Autodesk Fusion 360 part; units mm, degrees
(part 3 of 4)
  spline S773 degree 3 poles (-4.0952, -2.1163) (-4.5357, -1.9459) (-4.7047, -1.6279) (-4.6025, -1.1626) knots 0 0 0 0 1 1 1 1
  spline S774 degree 3 poles (-4.6025, -1.1626) (-4.3484, -0.6512) (-3.9899, -0.225) (-3.527, 0.1159) knots 0 0 0 0 1 1 1 1
  spline S775 degree 3 poles (-3.527, 0.1159) (-2.8898, 0.6509) (-2.1728, 1.0365) (-1.376, 1.2726) knots 0 0 0 0 1 1 1 1
  spline S776 degree 3 poles (-1.1325, 0.6232) (-2.2555, 0.3285) (-3.2092, -0.2533) (-3.9938, -1.122) knots 0 0 0 0 1 1 1 1
  spline S777 degree 3 poles (-3.9938, -1.122) (-4.1157, -1.269) (-4.1969, -1.4313) (-4.2373, -1.609) knots 0 0 0 0 1 1 1 1
  spline S778 degree 3 poles (-4.2373, -1.609) (-4.1708, -1.7027) (-4.0829, -1.7636) (-3.9735, -1.7916) knots 0 0 0 0 1 1 1 1
  spline S779 degree 3 poles (-3.9735, -1.7916) (-3.69, -1.836) (-3.4194, -1.7954) (-3.1617, -1.6699) knots 0 0 0 0 1 1 1 1
  spline S780 degree 3 poles (-3.1617, -1.6699) (-2.1944, -1.1222) (-1.3624, -0.4119) (-0.6657, 0.4609) knots 0 0 0 0 1 1 1 1
  spline S781 degree 3 poles (-0.6657, 0.4609) (-0.6205, 0.512) (-0.6138, 0.5594) (-0.6454, 0.6029) knots 0 0 0 0 1 1 1 1
  spline S782 degree 3 poles (-0.6454, 0.6029) (-0.8072, 0.6232) (-0.9695, 0.63) (-1.1325, 0.6232) knots 0 0 0 0 1 1 1 1
  spline S783 degree 3 poles (-14.7693, 1.2726) (-14.412, 1.3072) (-14.0737, 1.2463) (-13.7546, 1.09) knots 0 0 0 0 1 1 1 1
  spline S784 degree 3 poles (-13.7546, 1.09) (-13.6135, 0.9404) (-13.5932, 0.7713) (-13.6938, 0.5826) knots 0 0 0 0 1 1 1 1
  spline S785 degree 3 poles (-13.6938, 0.5826) (-13.9508, 0.1629) (-14.2688, -0.2092) (-14.6475, -0.5335) knots 0 0 0 0 1 1 1 1
  spline S786 degree 3 poles (-14.6475, -0.5335) (-15.0534, -0.8582) (-15.4592, -1.1828) (-15.8651, -1.5075) knots 0 0 0 0 1 1 1 1
  spline S787 degree 3 poles (-15.8651, -1.5075) (-16.2645, -1.7884) (-16.6974, -2.0049) (-17.1638, -2.1569) knots 0 0 0 0 1 1 1 1
  spline S788 degree 3 poles (-17.1638, -2.1569) (-17.7724, -2.2659) (-18.1377, -2.0224) (-18.2597, -1.4264) knots 0 0 0 0 1 1 1 1
  spline S789 degree 3 poles (-18.2597, -1.4264) (-18.1127, -0.9302) (-17.8422, -0.5108) (-17.4479, -0.1682) knots 0 0 0 0 1 1 1 1
  spline S790 degree 3 poles (-17.4479, -0.1682) (-16.6732, 0.537) (-15.7804, 1.0173) (-14.7693, 1.2726) knots 0 0 0 0 1 1 1 1
  spline S791 degree 3 poles (-14.8099, 0.5826) (-16.001, 0.2541) (-16.9818, -0.3953) (-17.7523, -1.3655) knots 0 0 0 0 1 1 1 1
  spline S792 degree 3 poles (-17.7523, -1.3655) (-17.916, -1.5781) (-17.8686, -1.7202) (-17.6103, -1.7916) knots 0 0 0 0 1 1 1 1
  spline S793 degree 3 poles (-17.6103, -1.7916) (-17.4615, -1.8187) (-17.3127, -1.8187) (-17.1638, -1.7916) knots 0 0 0 0 1 1 1 1
  spline S794 degree 3 poles (-17.1638, -1.7916) (-16.7697, -1.6554) (-16.4044, -1.4661) (-16.068, -1.2234) knots 0 0 0 0 1 1 1 1
  spline S795 degree 3 poles (-16.068, -1.2234) (-15.3561, -0.7146) (-14.7067, -0.1328) (-14.1199, 0.5218) knots 0 0 0 0 1 1 1 1
  spline S796 degree 3 poles (-14.1199, 0.5218) (-14.3424, 0.5806) (-14.5724, 0.6009) (-14.8099, 0.5826) knots 0 0 0 0 1 1 1 1
  spline S797 degree 3 poles (16.9284, 1.2726) (17.2847, 1.3072) (17.6232, 1.2463) (17.943, 1.09) knots 0 0 0 0 1 1 1 1
  spline S798 degree 3 poles (17.943, 1.09) (18.0185, 1.042) (18.0591, 0.9743) (18.0648, 0.887) knots 0 0 0 0 1 1 1 1
  spline S799 degree 3 poles (18.0648, 0.887) (18.0441, 0.7035) (17.9832, 0.5344) (17.8821, 0.3797) knots 0 0 0 0 1 1 1 1
  spline S800 degree 3 poles (17.8821, 0.3797) (17.6484, 0.0646) (17.3846, -0.2263) (17.0907, -0.4929) knots 0 0 0 0 1 1 1 1
  spline S801 degree 3 poles (17.0907, -0.4929) (16.6849, -0.8176) (16.279, -1.1423) (15.8731, -1.4669) knots 0 0 0 0 1 1 1 1
  spline S802 degree 3 poles (15.8731, -1.4669) (15.4003, -1.8421) (14.8658, -2.0788) (14.27, -2.1772) knots 0 0 0 0 1 1 1 1
  spline S803 degree 3 poles (14.27, -2.1772) (13.5646, -2.0944) (13.3211, -1.7156) (13.5395, -1.0408) knots 0 0 0 0 1 1 1 1
  spline S804 degree 3 poles (13.5395, -1.0408) (14.2059, -0.0906) (15.0785, 0.6061) (16.1572, 1.0494) knots 0 0 0 0 1 1 1 1
  spline S805 degree 3 poles (16.1572, 1.0494) (16.4142, 1.1438) (16.6711, 1.2182) (16.9284, 1.2726) knots 0 0 0 0 1 1 1 1
  spline S806 degree 3 poles (16.8878, 0.5826) (16.6881, 0.5291) (16.4852, 0.4682) (16.279, 0.4) knots 0 0 0 0 1 1 1 1
  spline S807 degree 3 poles (16.279, 0.4) (15.2944, -0.0031) (14.4896, -0.6321) (13.8642, -1.4872) knots 0 0 0 0 1 1 1 1
  spline S808 degree 3 poles (13.8642, -1.4872) (13.8341, -1.566) (13.8406, -1.6404) (13.8844, -1.7105) knots 0 0 0 0 1 1 1 1
  spline S809 degree 3 poles (13.8844, -1.7105) (14.1799, -1.8416) (14.4774, -1.8416) (14.7773, -1.7105) knots 0 0 0 0 1 1 1 1
  spline S810 degree 3 poles (14.7773, -1.7105) (15.1357, -1.5382) (15.4738, -1.3352) (15.792, -1.1017) knots 0 0 0 0 1 1 1 1
  spline S811 degree 3 poles (15.792, -1.1017) (16.4174, -0.6385) (16.9925, -0.1177) (17.5169, 0.4609) knots 0 0 0 0 1 1 1 1
  spline S812 degree 3 poles (17.5169, 0.4609) (17.5364, 0.4994) (17.5433, 0.5399) (17.5372, 0.5826) knots 0 0 0 0 1 1 1 1
  spline S813 degree 3 poles (17.5372, 0.5826) (17.3208, 0.5826) (17.1041, 0.5826) (16.8878, 0.5826) knots 0 0 0 0 1 1 1 1
  spline S814 degree 3 poles (25.6543, 1.1914) (25.6815, 1.0697) (25.7083, 0.9479) (25.7355, 0.8262) knots 0 0 0 0 1 1 1 1
  spline S815 degree 3 poles (25.7355, 0.8262) (25.7331, 0.8041) (25.7197, 0.7906) (25.6949, 0.7856) knots 0 0 0 0 1 1 1 1
  spline S816 degree 3 poles (25.6949, 0.7856) (25.6547, 0.9182) (25.6413, 1.0535) (25.6543, 1.1914) knots 0 0 0 0 1 1 1 1
  spline S817 degree 3 poles (10.8405, 1.0697) (10.9899, 1.0764) (11.1388, 1.0696) (11.287, 1.0494) knots 0 0 0 0 1 1 1 1
  spline S818 degree 3 poles (11.287, 1.0494) (11.4051, 1.044) (11.5, 0.9966) (11.5711, 0.9073) knots 0 0 0 0 1 1 1 1
  spline S819 degree 3 poles (11.5711, 0.9073) (11.4379, 0.7542) (11.2756, 0.6393) (11.084, 0.5623) knots 0 0 0 0 1 1 1 1
  spline S820 degree 3 poles (11.084, 0.5623) (10.6031, 0.3564) (10.1161, 0.3293) (9.6229, 0.4812) knots 0 0 0 0 1 1 1 1
  spline S821 degree 3 poles (9.6229, 0.4812) (9.9951, 0.7552) (10.401, 0.9514) (10.8405, 1.0697) knots 0 0 0 0 1 1 1 1
  spline S822 degree 3 poles (10.7999, 0.8667) (10.5828, 0.7924) (10.3665, 0.7045) (10.1506, 0.6029) knots 0 0 0 0 1 1 1 1
  spline S823 degree 3 poles (10.1506, 0.6029) (10.5418, 0.5621) (10.9071, 0.6432) (11.2464, 0.8464) knots 0 0 0 0 1 1 1 1
  spline S824 degree 3 poles (11.2464, 0.8464) (11.0982, 0.8667) (10.9493, 0.8734) (10.7999, 0.8667) knots 0 0 0 0 1 1 1 1
  spline S825 degree 3 poles (-1.3354, 0.7856) (-1.0645, 0.7923) (-0.7939, 0.7856) (-0.5237, 0.7653) knots 0 0 0 0 1 1 1 1
  spline S826 degree 3 poles (-0.5237, 0.7653) (-0.4472, 0.7565) (-0.3795, 0.7294) (-0.3207, 0.6841) knots 0 0 0 0 1 1 1 1
  spline S827 degree 3 poles (-0.3207, 0.6841) (-0.5262, 0.3433) (-0.763, 0.0254) (-1.031, -0.2697) knots 0 0 0 0 1 1 1 1
  spline S828 degree 3 poles (-1.031, -0.2697) (-1.5589, -0.7979) (-2.1339, -1.2646) (-2.7559, -1.6699) knots 0 0 0 0 1 1 1 1
  spline S829 degree 3 poles (-2.7559, -1.6699) (-3.1548, -1.9247) (-3.5877, -2.0194) (-4.0546, -1.954) knots 0 0 0 0 1 1 1 1
  spline S830 degree 3 poles (-4.0546, -1.954) (-4.485, -1.8081) (-4.5594, -1.5579) (-4.2779, -1.2031) knots 0 0 0 0 1 1 1 1
  spline S831 degree 3 poles (-4.2779, -1.2031) (-3.6287, -0.4193) (-2.8373, 0.1827) (-1.9036, 0.6029) knots 0 0 0 0 1 1 1 1
  spline S832 degree 3 poles (-1.9036, 0.6029) (-1.7093, 0.6647) (-1.52, 0.7256) (-1.3354, 0.7856) knots 0 0 0 0 1 1 1 1
  spline S833 degree 3 poles (-1.1325, 0.6232) (-2.2555, 0.3285) (-3.2092, -0.2533) (-3.9938, -1.122) knots 0 0 0 0 1 1 1 1
  spline S834 degree 3 poles (-3.9938, -1.122) (-4.1157, -1.269) (-4.1969, -1.4313) (-4.2373, -1.609) knots 0 0 0 0 1 1 1 1
  spline S835 degree 3 poles (-4.2373, -1.609) (-4.1708, -1.7027) (-4.0829, -1.7636) (-3.9735, -1.7916) knots 0 0 0 0 1 1 1 1
  spline S836 degree 3 poles (-3.9735, -1.7916) (-3.69, -1.836) (-3.4194, -1.7954) (-3.1617, -1.6699) knots 0 0 0 0 1 1 1 1
  spline S837 degree 3 poles (-3.1617, -1.6699) (-2.1944, -1.1222) (-1.3624, -0.4119) (-0.6657, 0.4609) knots 0 0 0 0 1 1 1 1
  spline S838 degree 3 poles (-0.6657, 0.4609) (-0.6205, 0.512) (-0.6138, 0.5594) (-0.6454, 0.6029) knots 0 0 0 0 1 1 1 1
  spline S839 degree 3 poles (-0.6454, 0.6029) (-0.8072, 0.6232) (-0.9695, 0.63) (-1.1325, 0.6232) knots 0 0 0 0 1 1 1 1
  spline S840 degree 3 poles (-14.7693, 0.7856) (-14.4789, 0.8022) (-14.1948, 0.7684) (-13.917, 0.6841) knots 0 0 0 0 1 1 1 1
  spline S841 degree 3 poles (-13.917, 0.6841) (-13.8984, 0.6673) (-13.8849, 0.647) (-13.8764, 0.6232) knots 0 0 0 0 1 1 1 1
  spline S842 degree 3 poles (-13.8764, 0.6232) (-13.9748, 0.4127) (-14.1033, 0.2233) (-14.262, 0.055) knots 0 0 0 0 1 1 1 1
  spline S843 degree 3 poles (-14.262, 0.055) (-14.9117, -0.568) (-15.6084, -1.1294) (-16.3521, -1.6293) knots 0 0 0 0 1 1 1 1
  spline S844 degree 3 poles (-16.3521, -1.6293) (-16.5772, -1.7486) (-16.8072, -1.8568) (-17.0421, -1.954) knots 0 0 0 0 1 1 1 1
  spline S845 degree 3 poles (-17.0421, -1.954) (-17.3741, -2.0677) (-17.6785, -2.0203) (-17.9553, -1.8119) knots 0 0 0 0 1 1 1 1
  spline S846 degree 3 poles (-17.9553, -1.8119) (-17.9989, -1.7483) (-18.0327, -1.6807) (-18.0567, -1.609) knots 0 0 0 0 1 1 1 1
  spline S847 degree 3 poles (-18.0567, -1.609) (-18.0071, -1.4691) (-17.9462, -1.3338) (-17.8741, -1.2031) knots 0 0 0 0 1 1 1 1
  spline S848 degree 3 poles (-17.8741, -1.2031) (-17.0428, -0.2152) (-16.0079, 0.4477) (-14.7693, 0.7856) knots 0 0 0 0 1 1 1 1
  spline S849 degree 3 poles (-14.8099, 0.5826) (-16.001, 0.2541) (-16.9818, -0.3953) (-17.7523, -1.3655) knots 0 0 0 0 1 1 1 1
  spline S850 degree 3 poles (-17.7523, -1.3655) (-17.916, -1.5781) (-17.8686, -1.7202) (-17.6103, -1.7916) knots 0 0 0 0 1 1 1 1
  spline S851 degree 3 poles (-17.6103, -1.7916) (-17.4615, -1.8187) (-17.3127, -1.8187) (-17.1638, -1.7916) knots 0 0 0 0 1 1 1 1
  spline S852 degree 3 poles (-17.1638, -1.7916) (-16.7697, -1.6554) (-16.4044, -1.4661) (-16.068, -1.2234) knots 0 0 0 0 1 1 1 1
  spline S853 degree 3 poles (-16.068, -1.2234) (-15.3561, -0.7146) (-14.7067, -0.1328) (-14.1199, 0.5218) knots 0 0 0 0 1 1 1 1
  spline S854 degree 3 poles (-14.1199, 0.5218) (-14.3424, 0.5806) (-14.5724, 0.6009) (-14.8099, 0.5826) knots 0 0 0 0 1 1 1 1
  spline S855 degree 3 poles (16.9284, 0.7856) (17.219, 0.8022) (17.5031, 0.7684) (17.7807, 0.6841) knots 0 0 0 0 1 1 1 1
  spline S856 degree 3 poles (17.7807, 0.6841) (17.7993, 0.6673) (17.8127, 0.647) (17.8213, 0.6232) knots 0 0 0 0 1 1 1 1
  spline S857 degree 3 poles (17.8213, 0.6232) (17.6435, 0.3168) (17.4272, 0.0395) (17.1719, -0.2088) knots 0 0 0 0 1 1 1 1
  spline S858 degree 3 poles (17.1719, -0.2088) (16.5708, -0.7425) (15.9348, -1.2295) (15.2644, -1.6699) knots 0 0 0 0 1 1 1 1
  spline S859 degree 3 poles (15.2644, -1.6699) (14.9036, -1.903) (14.5111, -2.0112) (14.0874, -1.9946) knots 0 0 0 0 1 1 1 1
  spline S860 degree 3 poles (14.0874, -1.9946) (13.6835, -1.9103) (13.5683, -1.687) (13.7424, -1.3249) knots 0 0 0 0 1 1 1 1
  spline S861 degree 3 poles (13.7424, -1.3249) (14.5614, -0.2557) (15.6235, 0.4478) (16.9284, 0.7856) knots 0 0 0 0 1 1 1 1
  spline S862 degree 3 poles (16.8878, 0.5826) (16.6881, 0.5291) (16.4852, 0.4682) (16.279, 0.4) knots 0 0 0 0 1 1 1 1
  spline S863 degree 3 poles (16.279, 0.4) (15.2944, -0.0031) (14.4896, -0.6321) (13.8642, -1.4872) knots 0 0 0 0 1 1 1 1
  spline S864 degree 3 poles (13.8642, -1.4872) (13.8341, -1.566) (13.8406, -1.6404) (13.8844, -1.7105) knots 0 0 0 0 1 1 1 1
  spline S865 degree 3 poles (13.8844, -1.7105) (14.1799, -1.8416) (14.4774, -1.8416) (14.7773, -1.7105) knots 0 0 0 0 1 1 1 1
  spline S866 degree 3 poles (14.7773, -1.7105) (15.1357, -1.5382) (15.4738, -1.3352) (15.792, -1.1017) knots 0 0 0 0 1 1 1 1
  spline S867 degree 3 poles (15.792, -1.1017) (16.4174, -0.6385) (16.9925, -0.1177) (17.5169, 0.4609) knots 0 0 0 0 1 1 1 1
  spline S868 degree 3 poles (17.5169, 0.4609) (17.5364, 0.4994) (17.5433, 0.5399) (17.5372, 0.5826) knots 0 0 0 0 1 1 1 1
  spline S869 degree 3 poles (17.5372, 0.5826) (17.3208, 0.5826) (17.1041, 0.5826) (16.8878, 0.5826) knots 0 0 0 0 1 1 1 1
  spline S870 degree 3 poles (-9.9802, -4.2877) (-9.9181, -4.2883) (-9.8978, -4.3154) (-9.9193, -4.3688) knots 0 0 0 0 1 1 1 1
  spline S871 degree 3 poles (-9.9193, -4.3688) (-10.4202, -5.0595) (-10.9816, -5.7021) (-11.6036, -6.2967) knots 0 0 0 0 1 1 1 1
  spline S872 degree 3 poles (-11.6036, -6.2967) (-11.793, -6.4319) (-11.9824, -6.5672) (-12.1718, -6.7025) knots 0 0 0 0 1 1 1 1
  spline S873 degree 3 poles (-12.1718, -6.7025) (-12.3381, -6.7873) (-12.514, -6.8347) (-12.6994, -6.8446) knots 0 0 0 0 1 1 1 1
  spline S874 degree 3 poles (-12.6994, -6.8446) (-12.6667, -6.6303) (-12.5787, -6.4409) (-12.4356, -6.2764) knots 0 0 0 0 1 1 1 1
  spline S875 degree 3 poles (-12.4356, -6.2764) (-12.1853, -6.0261) (-11.9351, -5.7758) (-11.6848, -5.5255) knots 0 0 0 0 1 1 1 1
  spline S876 degree 3 poles (-11.6848, -5.5255) (-11.1319, -5.087) (-10.5637, -4.6744) (-9.9802, -4.2877) knots 0 0 0 0 1 1 1 1
  spline S877 degree 3 poles (-11.8884, -6.4996) (-11.8875, -6.499) (-11.8867, -6.4984) (-11.8859, -6.4978) knots 0 0 0 0 1 1 1 1
  line L58 (-11.8859, -6.4978) -> (-11.8884, -6.4996)
extrude "Extrude1" add sketch "Sketch1" along normal blind 2.5 contours S0 L0 L1 L2 S1 S2 S3 S4 S5 L3 L4 S6 S7 L5 L6 S8 L7 S9 S10 S11 S12 S13 S14 L8 L9 S15 S16 L10 L11 S17 L12 S18 S19 S20 L13 L14 S21 S22 S23 L15 L16 S24 S25 L17 L18 S26 L19 L20 S27 S28 S29 S30 L21 S31 L22 L23 S32 S33 L24 S34 L25 L26 S35 S36 S37 L27 L28 S38 L29 S39 S40 S41 S42 S43 S44 S45 S46 L30 S47 S48 L31 L32 S49 S50 S51 S52 L33 L34 S53 S54 S55 L35 L36 S56 S57 L37 L38 S58 S59 S60 L39 L40 S61 S62 L41 S63 S64 S65 S66 S67 L42 L43 S68 S69 L44 L45 S70 L46 L47 S71 S72 S73 S74 L48 S75 S76 S77 L49 L50 S78 S79 S80 L51 L52 S81 S82 L53 L54 S83 S84 L55 S85 L56 L57 | S86 S87 S88 S89 S90 S91 S92 S93 S94 S95 S96 S97 S98 S99 S100 S101 S102 S103 S104 S105 S106 S107 S108 S109 S110 S111 S112 S113 S114 S115 S116 S117 S118 S119 S120 S121 S122 S123 S124 S125 S126 S127 S128 S129 S130 S131 S132 S133 S134 S135 S136 S137 S138 S139 S140 S141 S142 S143 S144 S145 S146 S147 S148 S149 S150 S151 S152 S153 S154 S155 S156 S157 S158 S159 S160 S161 S162 S163 S164 S165 S166 S167 S168 S169 S170 S171 S172 S173 S174 S175 S176 S177 S178 S179 S180 S181 S182 S183 S184 S185 S186 S187 S188 S189 S190 S191 S192 S193 S194 S195 S196 S197 S198 S199 S200 S201 S202 S203 S204 S205 S206 S207 S208 S209 S210 S211 S212 | S213 S214 S215 S216 S217 S415 S416 S417 S418 S419 S515 S516 S517 S518 S519 S527 S528 S529 S530 S531 S537 S538 S539 S540 S541 | S218 S219 S220 S221 S222 S223 S224 S225 S226 S227 S228 S229 S230 S231 S232 S420 S421 S422 S423 S424 S425 S426 S427 S428 S429 S430 S431 S432 S433 S434 S560 S561 S562 S563 S564 S565 S566 S567 S568 S569 S570 S571 S572 S573 S574 | S233 S234 S235 S236 S237 S435 S436 S437 S438 S439 S752 S753 S754 S755 S756 | S238 S239 S240 S440 S441 S442 S722 S723 S724 S765 S766 S767 S822 S823 S824 | S241 S242 S243 S244 S245 S246 S247 S443 S444 S445 S446 S447 S448 S449 S725 S726 S727 S728 S729 S730 S731 S776 S777 S778 S779 S780 S781 S782 S833 S834 S835 S836 S837 S838 S839 | S248 S249 S250 S251 S252 S253 S450 S451 S452 S453 S454 S455 S732 S733 S734 S735 S736 S737 S791 S792 S793 S794 S795 S796 S849 S850 S851 S852 S853 S854 | S254 S255 S256 S257 S258 S259 S260 S261 S456 S457 S458 S459 S460 S461 S462 S463 S738 S739 S740 S741 S742 S743 S744 S745 S806 S807 S808 S809 S810 S811 S812 S813 S862 S863 S864 S865 S866 S867 S868 S869 | S262 S263 S264 S265 S266 S464 S465 S466 S467 S468 | S267 S268 S269 S270 S271 S272 S273 S274 S275 S276 S277 S278 S279 S280 S281 S282 S283 S284 S285 S286 S287 S288 S289 S290 S291 S292 S293 S294 S295 S296 S297 S298 S299 S300 S301 S302 S303 S304 S305 S306 S307 S308 S309 S310 S311 S312 S313 S314 S315 S316 S317 S318 S319 S320 S321 S322 S323 S324 S325 S326 S327 S328 S329 S330 S331 S332 S333 S334 S335 S336 S337 S338 S339 S340 S341 S342 S343 S344 S345 S346 S347 S348 S349 S350 S351 S352 S353 S354 S355 S356 S357 S358 S359 S360 S361 S362 S363 S364 S365 S366 S367 S368 S369 S370 S371 S372 S373 S374 S375 S376 S377 S378 S379 S380 S381 S382 S383 S384 S385 S386 S387 S388 S389 S390 S391 S392 S393 S394 S395 S396 S397 S398 S399 S400 S401 S402 S403 S404 S405 S406 S407 S408 S409 S410 S411 S412 S413 S414 | S469 S470 S471 S472 S473 S474 S475 S476 S477 S478 S479 S480 S481 S482 S483 S484 S485 S486 S487 S488 S489 S490 S491 S492 S493 S494 S495 S496 S497 S498 S499 S500 S501 S502 S503 S504 S505 S506 S507 S508 S509 S510 S511 S512 S513 S514 | S520 S521 S522 S523 S524 S525 S526 | S532 S533 S534 S535 S536 | S542 S543 S544 S545 | S546 S547 S548 S549 S550 S551 S552 S553 S554 S555 S556 S557 S558 S559 | S575 S576 S814 S815 S816 | S575 S576 S577 S578 S579 S580 S581 S582 S583 S584 S585 S586 S587 S588 S589 S590 S591 S592 S593 S594 S595 S596 S597 S598 S599 S600 S601 S602 S603 S604 S605 S606 S607 S608 S609 S610 S611 S612 S613 S614 S615 S616 S617 S618 S619 S620 S621 S622 S623 S624 S625 S626 S627 S628 S629 S630 S631 S632 S633 S634 S635 S636 S637 S638 S639 S640 S641 S642 S643 S644 S645 S646 S647 S648 S649 S650 S651 S652 S653 S654 S655 S656 S657 S658 S659 S660 S661 S662 S663 S664 S665 S666 S667 S668 S669 S670 S671 S672 S673 S674 S675 S676 S677 S678 S679 S680 S681 S682 S683 S684 S685 S686 S687 S688 S689 S690 S691 S692 S693 S694 S695 S696 S697 S698 S699 S700 S701 S702 S703 S704 S705 S706 S707 S708 S709 S710 S711 S712 S713 S714 S715 S716 S717 S718 S719 S720 S721 S815 S816 | S746 S757 S758 S759 | S746 S747 S748 S749 S750 S751 S759 | S760 S761 S762 S763 S764 | S768 S769 S770 S771 S772 S773 S774 S775 | S783 S784 S785 S786 S787 S788 S789 S790 | S797 S798 S799 S800 S801 S802 S803 S804 S805 | S817 S818 S819 S820 S821 | S825 S826 S827 S828 S829 S830 S831 S832 | S840 S841 S842 S843 S844 S845 S846 S847 S848 | S855 S856 S857 S858 S859 S860 S861 | S870 S871 S872 S873 S874 S875 S876 S877 L58 makes body 1
move_body "Move1" bodies 1 to x (1, 0, 0) y (0, 1, 0) z (0, 0, 1) at (0, 0, -2.5)
extrude "Extrude2" add sketch "Sketch1" along normal blind 2 contours S469 S470 S471 S472 S473 S474 S475 S476 S477 S478 S479 S480 S481 S482 S483 S484 S485 S486 S487 S488 S489 S490 S491 S492 S493 S494 S495 S496 S497 S498 S499 S500 S501 S502 S503 S504 S505 S506 S507 S508 S509 S510 S511 S512 S513 S514 | S575 S576 S577 S578 S579 S580 S581 S582 S583 S584 S585 S586 S587 S588 S589 S590 S591 S592 S593 S594 S595 S596 S597 S598 S599 S600 S601 S602 S603 S604 S605 S606 S607 S608 S609 S610 S611 S612 S613 S614 S615 S616 S617 S618 S619 S620 S621 S622 S623 S624 S625 S626 S627 S628 S629 S630 S631 S632 S633 S634 S635 S636 S637 S638 S639 S640 S641 S642 S643 S644 S645 S646 S647 S648 S649 S650 S651 S652 S653 S654 S655 S656 S657 S658 S659 S660 S661 S662 S663 S664 S665 S666 S667 S668 S669 S670 S671 S672 S673 S674 S675 S676 S677 S678 S679 S680 S681 S682 S683 S684 S685 S686 S687 S688 S689 S690 S691 S692 S693 S694 S695 S696 S697 S698 S699 S700 S701 S702 S703 S704 S705 S706 S707 S708 S709 S710 S711 S712 S713 S714 S715 S716 S717 S718 S719 S720 S721 S815 S816 bodies 1
sketch "Sketch2" plane through (0, 0, 0) normal (0, 0, 1) x (1, 0, 0)
  circle A0 centre (36, -1) radius 4
  dimension "d5" = 8
  measures "d5" diameter of A0
extrude "Extrude3" add sketch "Sketch2" against normal blind 2.5 bodies 1
sketch "Sketch3" plane through (0, 0, 0) normal (0, 0, 1) x (-1, 0, 0)
  spline S0 degree 3 poles (-33.3647, -2.0092) (-33.0581, -2.2998) (-32.6822, -2.565) (-32.2357, -2.7561) knots -0.773716 -0.773716 -0.773716 -0.773716 0 0 0 0
  spline S1 degree 3 poles (-32.2357, -2.7561) (-32.1732, -2.8929) (-32.1022, -3.0293) (-32.0218, -3.1648) knots -1 -1 -1 -1 0 0 0 0
  spline S2 degree 3 poles (-32.0218, -3.1648) (-31.3201, -4.3441) (-30.2162, -4.9191) (-29.2681, -5.1795) knots -1 -1 -1 -1 0 0 0 0
  line L0 (-29.2681, -5.1795) -> (-29.223, -5.1916)
  line L1 (-29.223, -5.1916) -> (-29.1654, -5.2065)
  spline S3 degree 3 poles (-29.1654, -5.2065) (-28.8951, -5.2734) (-28.626, -5.3065) (-28.365, -5.3111) knots -1 -1 -1 -1 0 0 0 0
  line L2 (-28.365, -5.3111) -> (-28.3094, -5.3117)
  spline S4 degree 3 poles (-28.3094, -5.3117) (-27.6787, -5.313) (-27.0557, -5.231) (-26.451, -5.0601) knots -1 -1 -1 -1 0 0 0 0
  spline S5 degree 3 poles (-26.451, -5.0601) (-25.9124, -5.2986) (-25.3605, -5.4125) (-24.8398, -5.4441) knots -1 -1 -1 -1 0 0 0 0
  line L3 (-24.8398, -5.4441) -> (-24.7663, -5.448)
  line L4 (-24.7663, -5.448) -> (-24.7241, -5.4497)
  spline S6 degree 3 poles (-24.7241, -5.4497) (-24.5277, -5.4565) (-24.3442, -5.4463) (-24.1774, -5.4264) knots -1 -1 -1 -1 0 0 0 0
  line L5 (-24.1774, -5.4264) -> (-24.1417, -5.422)
  spline S7 degree 3 poles (-24.1417, -5.422) (-23.7594, -5.3726) (-23.3835, -5.2965) (-23.0154, -5.1941) knots -1 -1 -1 -1 0 0 0 0
  spline S8 degree 3 poles (-23.0154, -5.1941) (-22.3624, -5.406) (-21.4931, -5.5135) (-20.5645, -5.1964) knots -1 -1 -1 -1 0 0 0 0
  spline S9 degree 3 poles (-20.5645, -5.1964) (-20.295, -5.1043) (-20.051, -4.9869) (-19.8311, -4.8523) knots -1 -1 -1 -1 0 0 0 0
  spline S10 degree 3 poles (-19.8311, -4.8523) (-19.6659, -4.9416) (-19.4966, -5.0207) (-19.3246, -5.0901) knots -1 -1 -1 -1 0 0 0 0
  line L6 (-19.3246, -5.0901) -> (-19.1642, -5.1546)
  line L7 (-19.1642, -5.1546) -> (-18.9978, -5.2007)
  spline S11 degree 3 poles (-18.9978, -5.2007) (-17.9994, -5.4769) (-16.9738, -5.5254) (-15.9543, -5.346) knots -1 -1 -1 -1 0 0 0 0
  line L8 (-15.9543, -5.346) -> (-15.8313, -5.3244)
  line L9 (-15.8313, -5.3244) -> (-15.7108, -5.2928)
  spline S12 degree 3 poles (-15.7108, -5.2928) (-15.1775, -5.1532) (-14.6637, -4.9752) (-14.1702, -4.7588) knots -1 -1 -1 -1 0 0 0 0
  spline S13 degree 3 poles (-14.1702, -4.7588) (-12.8633, -5.6981) (-11.293, -5.9769) (-9.7098, -5.5886) knots -1 -1 -1 -1 0 0 0 0
  line L10 (-9.7098, -5.5886) -> (-9.672, -5.5794)
  line L11 (-9.672, -5.5794) -> (-9.6347, -5.5692)
  spline S14 degree 3 poles (-9.6347, -5.5692) (-9.0085, -5.3986) (-8.4135, -5.1588) (-7.8558, -4.8512) knots -1 -1 -1 -1 0 0 0 0
  spline S15 degree 3 poles (-7.8558, -4.8512) (-7.8335, -5.0337) (-7.8023, -5.2143) (-7.7621, -5.3924) knots -1 -1 -1 -1 0 0 0 0
  spline S16 degree 3 poles (-7.7621, -5.3924) (-7.6785, -5.7617) (-7.5348, -6.1216) (-7.3319, -6.4552) knots -1 -1 -1 -1 0 0 0 0
  line L12 (-7.3319, -6.4552) -> (-7.312, -6.4874)
  line L13 (-7.312, -6.4874) -> (-7.2909, -6.5213)
  spline S17 degree 3 poles (-7.2909, -6.5213) (-6.8371, -7.2358) (-6.0538, -8.0631) (-4.8203, -8.3805) knots -1 -1 -1 -1 0 0 0 0
  spline S18 degree 3 poles (-4.8203, -8.3805) (-3.5755, -8.7007) (-2.4822, -8.3441) (-1.7475, -7.945) knots -1 -1 -1 -1 0 0 0 0
  spline S19 degree 3 poles (-1.7475, -7.945) (-1.4187, -7.7663) (-1.1579, -7.5569) (-0.9577, -7.3625) knots -1 -1 -1 -1 0 0 0 0
  line L14 (-0.9577, -7.3625) -> (-0.9184, -7.3239)
  spline S20 degree 3 poles (-0.9184, -7.3239) (-0.8098, -7.2152) (-0.7011, -7.1065) (-0.5924, -6.9978) knots -1 -1 -1 -1 0 0 0 0
  line L15 (-0.5924, -6.9978) -> (-0.1573, -6.5627)
  line L16 (-0.1573, -6.5627) -> (-0.0598, -6.4431)
  spline S21 degree 3 poles (-0.0598, -6.4431) (0.1999, -6.1247) (0.4568, -5.8048) (0.7109, -5.4834) knots -1 -1 -1 -1 0 0 0 0
  spline S22 degree 3 poles (0.7109, -5.4834) (1.4698, -5.5072) (2.2264, -5.4039) (2.9669, -5.1745) knots -1 -1 -1 -1 0 0 0 0
  line L17 (2.9669, -5.1745) -> (3.0332, -5.1539)
  line L18 (3.0332, -5.1539) -> (3.0985, -5.1304)
  spline S23 degree 3 poles (3.0985, -5.1304) (3.2942, -5.0598) (3.487, -4.9839) (3.677, -4.9028) knots -1 -1 -1 -1 0 0 0 0
  spline S24 degree 3 poles (3.677, -4.9028) (3.7986, -4.9737) (3.921, -5.0355) (4.0426, -5.0886) knots -1 -1 -1 -1 0 0 0 0
  spline S25 degree 3 poles (4.0426, -5.0886) (4.8296, -5.4328) (5.8678, -5.6394) (6.985, -5.3047) knots -1 -1 -1 -1 0 0 0 0
  spline S26 degree 3 poles (6.985, -5.3047) (7.0121, -5.2966) (7.0389, -5.2882) (7.0656, -5.2796) knots -1 -1 -1 -1 0 0 0 0
  spline S27 degree 3 poles (7.0656, -5.2796) (7.3065, -5.3766) (7.5435, -5.4451) (7.7656, -5.4916) knots -1 -1 -1 -1 0 0 0 0
  spline S28 degree 3 poles (7.7656, -5.4916) (8.3289, -5.6096) (8.8543, -5.5745) (9.2942, -5.4714) knots -1 -1 -1 -1 0 0 0 0
  line L19 (9.2942, -5.4714) -> (9.3365, -5.4613)
  spline S29 degree 3 poles (9.3365, -5.4613) (9.8393, -5.3371) (10.3204, -5.1508) (10.7746, -4.9061) knots -1 -1 -1 -1 0 0 0 0
  line L20 (10.7746, -4.9061) -> (10.8053, -4.8895)
  line L21 (10.8053, -4.8895) -> (10.8356, -4.8723)
  spline S30 degree 3 poles (10.8356, -4.8723) (11.016, -4.7697) (11.1926, -4.6617) (11.3653, -4.5483) knots -1 -1 -1 -1 0 0 0 0
  spline S31 degree 3 poles (11.3653, -4.5483) (11.5266, -4.6643) (11.6952, -4.7703) (11.8702, -4.8661) knots -1 -1 -1 -1 0 0 0 0
  line L22 (11.8702, -4.8661) -> (11.9101, -4.8877)
  line L23 (11.9101, -4.8877) -> (11.9485, -4.908)
  spline S32 degree 3 poles (11.9485, -4.908) (12.1403, -5.0077) (12.3281, -5.083) (12.505, -5.1397) knots -1 -1 -1 -1 0 0 0 0
  spline S33 degree 3 poles (12.505, -5.1397) (12.5953, -5.1686) (12.686, -5.1955) (12.7769, -5.2205) knots -1 -1 -1 -1 0 0 0 0
  spline S34 degree 3 poles (12.7769, -5.2205) (12.6296, -5.4157) (12.5074, -5.614) (12.4073, -5.8054) knots -1 -1 -1 -1 0 0 0 0
  spline S35 degree 3 poles (12.4073, -5.8054) (12.2329, -6.1392) (12.1242, -6.4791) (12.0651, -6.8032) knots -1 -1 -1 -1 0 0 0 0
  spline S36 degree 3 poles (12.0651, -6.8032) (11.8163, -8.1682) (12.1523, -9.5077) (13.0154, -10.5937) knots -1 -1 -1 -1 0 0 0 0
  line L24 (13.0154, -10.5937) -> (13.1095, -10.7122)
  line L25 (13.1095, -10.7122) -> (13.215, -10.8207)
  line L26 (13.215, -10.8207) -> (13.2633, -10.87)
  spline S37 degree 3 poles (13.2633, -10.87) (14.2829, -11.8983) (15.5656, -12.5271) (17.0116, -12.697) knots -1 -1 -1 -1 0 0 0 0
  line L27 (17.0116, -12.697) -> (17.1886, -12.7178)
  line L28 (17.1886, -12.7178) -> (18.5296, -12.7178)
  spline S38 degree 3 poles (18.5296, -12.7178) (18.7199, -12.7178) (18.9214, -12.7031) (19.1303, -12.6684) knots -1 -1 -1 -1 0 0 0 0
  line L29 (19.1303, -12.6684) -> (19.1721, -12.6612)
  spline S39 degree 3 poles (19.1721, -12.6612) (19.9708, -12.519) (20.7386, -12.2804) (21.4699, -11.9478) knots -1 -1 -1 -1 0 0 0 0
  spline S40 degree 3 poles (21.4699, -11.9478) (22.2378, -12.0846) (23.0183, -12.1123) (23.8029, -12.0325) knots -1 -1 -1 -1 0 0 0 0
  line L30 (23.8029, -12.0325) -> (23.8069, -12.0321)
  line L31 (23.8069, -12.0321) -> (23.8109, -12.0317)
  spline S41 degree 3 poles (23.8109, -12.0317) (24.8876, -11.9194) (25.9553, -11.5669) (26.8945, -10.8753) knots -1 -1 -1 -1 0 0 0 0
  spline S42 degree 3 poles (26.8945, -10.8753) (27.8342, -10.1832) (28.4879, -9.2675) (28.9131, -8.2699) knots -1 -1 -1 -1 0 0 0 0
  line L32 (28.9131, -8.2699) -> (28.9707, -8.1349)
  line L33 (28.9707, -8.1349) -> (29.015, -7.995)
  spline S43 degree 3 poles (29.015, -7.995) (29.3472, -6.9455) (29.4617, -5.7423) (29.0788, -4.5231) knots -1 -1 -1 -1 0 0 0 0
  spline S44 degree 3 poles (29.0788, -4.5231) (28.9939, -4.2524) (28.8892, -3.9964) (28.768, -3.7547) knots -1 -1 -1 -1 0 0 0 0
  spline S45 degree 3 poles (28.768, -3.7547) (28.7892, -3.718) (28.8105, -3.6813) (28.8316, -3.6446) knots -1 -1 -1 -1 0 0 0 0
  line L34 (28.8316, -3.6446) -> (28.8667, -3.5837)
  line L35 (28.8667, -3.5837) -> (28.8989, -3.5214)
  spline S46 degree 3 poles (28.8989, -3.5214) (29.2125, -2.914) (29.538, -2.3142) (29.8752, -1.722) knots -1 -1 -1 -1 0 0 0 0
  spline S47 degree 3 poles (29.8752, -1.722) (30.4923, -1.8894) (31.2617, -1.949) (32.0873, -1.6748) knots -1 -1 -1 -1 0 0 0 0
  spline S48 degree 3 poles (32.0873, -1.6748) (33.1666, -1.3164) (33.8311, -0.5581) (34.2072, 0.0914) knots -1 -1 -1 -1 0 0 0 0
  line L36 (34.2072, 0.0914) -> (34.2428, 0.1539)
  spline S49 degree 3 poles (34.2428, 0.1539) (34.5131, 0.6391) (34.6399, 1.1377) (34.6769, 1.5881) knots -1 -1 -1 -1 0 0 0 0
  spline S50 degree 3 poles (34.6769, 1.5881) (34.729, 2.2215) (34.6825, 2.854) (34.537, 3.4741) knots -1 -1 -1 -1 0 0 0 0
  spline S51 degree 3 poles (34.537, 3.4741) (34.4452, 3.8656) (34.2876, 4.2408) (34.0693, 4.5827) knots -1 -1 -1 -1 0 0 0 0
  spline S52 degree 3 poles (34.0693, 4.5827) (33.0924, 6.1128) (31.5585, 6.9767) (29.7849, 7.0826) knots -1 -1 -1 -1 0 0 0 0
  line L37 (29.7849, 7.0826) -> (29.618, 7.0926)
  line L38 (29.618, 7.0926) -> (29.451, 7.0843)
  spline S53 degree 3 poles (29.451, 7.0843) (28.1898, 7.0211) (27.0239, 6.612) (26.0235, 5.8808) knots -1 -1 -1 -1 0 0 0 0
  line L39 (26.0235, 5.8808) -> (25.9385, 5.9284)
  line L40 (25.9385, 5.9284) -> (25.7467, 6.0039)
  spline S54 degree 3 poles (25.7467, 6.0039) (23.8226, 6.7614) (21.8163, 6.8437) (19.9578, 6.0404) knots -1 -1 -1 -1 0 0 0 0
  spline S55 degree 3 poles (19.9578, 6.0404) (19.4621, 6.3149) (18.9423, 6.492) (18.4342, 6.5979) knots -1 -1 -1 -1 0 0 0 0
  line L41 (18.4342, 6.5979) -> (18.2993, 6.626)
  line L42 (18.2993, 6.626) -> (18.1624, 6.6418)
  spline S56 degree 3 poles (18.1624, 6.6418) (17.7496, 6.6895) (17.3371, 6.6975) (16.9287, 6.6644) knots -1 -1 -1 -1 0 0 0 0
  spline S57 degree 3 poles (16.9287, 6.6644) (16.9595, 7.1724) (16.9174, 7.6941) (16.7998, 8.221) knots -1 -1 -1 -1 0 0 0 0
  spline S58 degree 3 poles (16.7998, 8.221) (16.7448, 8.4674) (16.6574, 8.7371) (16.5217, 9.0129) knots -1 -1 -1 -1 0 0 0 0
  spline S59 degree 3 poles (16.5217, 9.0129) (15.9537, 10.1675) (14.941, 10.9952) (13.6596, 11.2964) knots -1 -1 -1 -1 0 0 0 0
  spline S60 degree 3 poles (13.6596, 11.2964) (13.3343, 11.3729) (13.0495, 11.3902) (12.8404, 11.3902) knots -1 -1 -1 -1 0 0 0 0
  line L43 (12.8404, 11.3902) -> (12.4606, 11.3902)
  spline S61 degree 3 poles (12.4606, 11.3902) (12.1496, 11.3902) (11.7998, 11.3511) (11.4328, 11.2431) knots -1 -1 -1 -1 0 0 0 0
  spline S62 degree 3 poles (11.4328, 11.2431) (10.6783, 11.0211) (9.9808, 10.6718) (9.352, 10.2087) knots -1 -1 -1 -1 0 0 0 0
  line L44 (9.352, 10.2087) -> (9.2488, 10.1326)
  line L45 (9.2488, 10.1326) -> (9.1522, 10.0482)
  spline S63 degree 3 poles (9.1522, 10.0482) (7.8863, 8.94) (6.8039, 7.6764) (5.9117, 6.2637) knots -1 -1 -1 -1 0 0 0 0
  spline S64 degree 3 poles (5.9117, 6.2637) (5.9044, 6.2599) (5.897, 6.2561) (5.8897, 6.2522) knots -1 -1 -1 -1 0 0 0 0
  spline S65 degree 3 poles (5.8897, 6.2522) (5.4048, 6.461) (4.8971, 6.5878) (4.3865, 6.6438) knots -1 -1 -1 -1 0 0 0 0
  line L46 (4.3865, 6.6438) -> (4.3, 6.6533)
  line L47 (4.3, 6.6533) -> (4.213, 6.6578)
  spline S66 degree 3 poles (4.213, 6.6578) (3.4266, 6.6988) (2.6487, 6.6088) (1.8986, 6.3792) knots -1 -1 -1 -1 0 0 0 0
  line L48 (1.8986, 6.3792) -> (1.8911, 6.3814)
  line L49 (1.8911, 6.3814) -> (1.6858, 6.4404)
  line L50 (1.6858, 6.4404) -> (1.4742, 6.47)
  spline S67 degree 3 poles (1.4742, 6.47) (0.2935, 6.6357) (-0.8662, 6.4685) (-1.9401, 5.9861) knots -1 -1 -1 -1 0 0 0 0
  spline S68 degree 3 poles (-1.9401, 5.9861) (-1.9493, 5.9928) (-1.9586, 5.9996) (-1.968, 6.0062) knots -1 -1 -1 -1 0 0 0 0
  spline S69 degree 3 poles (-1.968, 6.0062) (-2.8406, 6.6275) (-3.8027, 6.8123) (-4.6218, 6.8038) knots -1 -1 -1 -1 0 0 0 0
  line L51 (-4.6218, 6.8038) -> (-4.7783, 6.8022)
  line L52 (-4.7783, 6.8022) -> (-4.9338, 6.7845)
  spline S70 degree 3 poles (-4.9338, 6.7845) (-5.6161, 6.707) (-6.2803, 6.5562) (-6.922, 6.3326) knots -1 -1 -1 -1 0 0 0 0
  spline S71 degree 3 poles (-6.922, 6.3326) (-7.6135, 6.5812) (-8.3392, 6.6769) (-9.0657, 6.6378) knots -1 -1 -1 -1 0 0 0 0
  spline S72 degree 3 poles (-9.0657, 6.6378) (-10.0264, 6.5894) (-10.959, 6.4139) (-11.8556, 6.1104) knots -1 -1 -1 -1 0 0 0 0
  spline S73 degree 3 poles (-11.8556, 6.1104) (-12.1742, 6.277) (-12.5062, 6.4075) (-12.8455, 6.5043) knots -1 -1 -1 -1 0 0 0 0
  line L53 (-12.8455, 6.5043) -> (-12.9761, 6.5416)
  line L54 (-12.9761, 6.5416) -> (-13.1093, 6.5671)
  spline S74 degree 3 poles (-13.1093, 6.5671) (-14.0736, 6.7516) (-15.0484, 6.7163) (-15.9868, 6.438) knots -1 -1 -1 -1 0 0 0 0
  spline S75 degree 3 poles (-15.9868, 6.438) (-16.4758, 6.5698) (-16.9726, 6.6187) (-17.4605, 6.5984) knots -1 -1 -1 -1 0 0 0 0
  line L55 (-17.4605, 6.5984) -> (-17.5047, 6.5966)
  spline S76 degree 3 poles (-17.5047, 6.5966) (-18.8116, 7.0734) (-20.2146, 6.6354) (-21.058, 5.8602) knots -1 -1 -1 -1 0 0 0 0
  spline S77 degree 3 poles (-21.058, 5.8602) (-22.3924, 6.8462) (-24.125, 6.7788) (-25.3735, 5.9051) knots -1 -1 -1 -1 0 0 0 0
  spline S78 degree 3 poles (-25.3735, 5.9051) (-25.4145, 5.9271) (-25.4542, 5.9479) (-25.4936, 5.9673) knots -1 -1 -1 -1 0 0 0 0
  spline S79 degree 3 poles (-25.4936, 5.9673) (-26.8147, 6.6195) (-28.2575, 6.6903) (-29.6256, 6.2058) knots -1 -1 -1 -1 0 0 0 0
  spline S80 degree 3 poles (-29.6256, 6.2058) (-29.6285, 6.2048) (-29.6313, 6.2038) (-29.6338, 6.2029) knots -1 -1 -1 -1 0 0 0 0
  spline S81 degree 3 poles (-29.6338, 6.2029) (-29.6366, 6.202) (-29.639, 6.2011) (-29.6415, 6.2002) knots -1 -1 -1 -1 0 0 0 0
  spline S82 degree 3 poles (-29.6415, 6.2002) (-31.0231, 5.7123) (-32.2369, 4.9419) (-33.2442, 3.8992) knots -1 -1 -1 -1 -0.114858 -0.114858 -0.114858 -0.114858
  arc A0 (-33.2442, 3.8992) -> (-33.3647, -2.0092) centre (-36, 1) ccw
  spline S83 degree 3 poles (21.0398, -8.3345) (20.261, -8.8494) (19.4155, -9.1876) (18.5032, -9.3492) knots 0 0 0 0 1 1 1 1
  spline S84 degree 3 poles (18.5032, -9.3492) (17.6562, -9.4316) (16.858, -9.276) (16.1086, -8.8824) knots 0 0 0 0 1 1 1 1
  spline S85 degree 3 poles (16.1086, -8.8824) (15.7821, -8.6642) (15.5454, -8.3733) (15.3984, -8.0098) knots 0 0 0 0 1 1 1 1
  spline S86 degree 3 poles (15.3984, -8.0098) (15.3446, -7.5901) (15.5273, -7.394) (15.9463, -7.4213) knots 0 0 0 0 1 1 1 1
  spline S87 degree 3 poles (15.9463, -7.4213) (16.0104, -7.45) (16.0713, -7.4838) (16.1289, -7.5228) knots 0 0 0 0 1 1 1 1
  spline S88 degree 3 poles (16.1289, -7.5228) (16.3363, -8.0225) (16.7083, -8.3133) (17.245, -8.3954) knots 0 0 0 0 1 1 1 1
  spline S89 degree 3 poles (17.245, -8.3954) (18.2437, -8.5762) (19.1772, -8.4071) (20.0454, -7.8881) knots 0 0 0 0 1 1 1 1
  spline S90 degree 3 poles (20.0454, -7.8881) (18.6024, -6.8964) (17.8854, -5.5164) (17.8944, -3.7483) knots 0 0 0 0 1 1 1 1
  spline S91 degree 3 poles (17.8944, -3.7483) (17.9234, -1.9636) (18.4442, -0.3401) (19.4569, 1.122) knots 0 0 0 0 1 1 1 1
  spline S92 degree 3 poles (19.4569, 1.122) (20.0686, 1.91) (20.8465, 2.4579) (21.7906, 2.7657) knots 0 0 0 0 1 1 1 1
  spline S93 degree 3 poles (21.7906, 2.7657) (22.926, 3.1064) (23.9677, 2.9305) (24.9157, 2.2381) knots 0 0 0 0 1 1 1 1
  spline S94 degree 3 poles (24.9157, 2.2381) (25.5232, 1.656) (25.7599, 0.9457) (25.626, 0.1073) knots 0 0 0 0 1 1 1 1
  spline S95 degree 3 poles (25.626, 0.1073) (25.4125, -0.6474) (24.9186, -1.087) (24.1446, -1.2117) knots 0 0 0 0 1 1 1 1
  spline S96 degree 3 poles (24.1446, -1.2117) (23.6207, -1.2236) (23.1066, -1.156) (22.6023, -1.0088) knots 0 0 0 0 1 1 1 1
  spline S97 degree 3 poles (22.6023, -1.0088) (22.3358, -0.9581) (22.1397, -0.816) (22.0138, -0.5826) knots 0 0 0 0 1 1 1 1
  spline S98 degree 3 poles (22.0138, -0.5826) (21.9865, -0.1636) (22.1826, 0.019) (22.6023, -0.0347) knots 0 0 0 0 1 1 1 1
  spline S99 degree 3 poles (22.6023, -0.0347) (23.1335, -0.2942) (23.6882, -0.3754) (24.2664, -0.2782) knots 0 0 0 0 1 1 1 1
  spline S100 degree 3 poles (24.2664, -0.2782) (24.6176, -0.1035) (24.7799, 0.1806) (24.7534, 0.5741) knots 0 0 0 0 1 1 1 1
  spline S101 degree 3 poles (24.7534, 0.5741) (24.7601, 1.0409) (24.5707, 1.4061) (24.1852, 1.6699) knots 0 0 0 0 1 1 1 1
  spline S102 degree 3 poles (24.1852, 1.6699) (23.6603, 1.9874) (23.0921, 2.0957) (22.4806, 1.9946) knots 0 0 0 0 1 1 1 1
  spline S103 degree 3 poles (22.4806, 1.9946) (21.5608, 1.8425) (20.81, 1.4028) (20.2281, 0.6755) knots 0 0 0 0 1 1 1 1
  spline S104 degree 3 poles (20.2281, 0.6755) (19.4037, -0.4439) (18.9302, -1.702) (18.8076, -3.099) knots 0 0 0 0 1 1 1 1
  spline S105 degree 3 poles (18.8076, -3.099) (18.6631, -4.1951) (18.8796, -5.2098) (19.4569, -6.1429) knots 0 0 0 0 1 1 1 1
  spline S106 degree 3 poles (19.4569, -6.1429) (19.8338, -6.6553) (20.3072, -7.0476) (20.8774, -7.3199) knots 0 0 0 0 1 1 1 1
  spline S107 degree 3 poles (20.8774, -7.3199) (21.5825, -6.7128) (22.198, -6.0296) (22.7241, -5.2703) knots 0 0 0 0 1 1 1 1
  spline S108 degree 3 poles (22.7241, -5.2703) (22.397, -5.3207) (22.0859, -5.429) (21.7906, -5.595) knots 0 0 0 0 1 1 1 1
  spline S109 degree 3 poles (21.7906, -5.595) (21.4151, -5.8621) (21.0633, -6.1598) (20.7354, -6.4879) knots 0 0 0 0 1 1 1 1
  spline S110 degree 3 poles (20.7354, -6.4879) (20.4696, -6.6428) (20.2464, -6.5955) (20.0657, -6.3458) knots 0 0 0 0 1 1 1 1
  spline S111 degree 3 poles (20.0657, -6.3458) (20.0235, -6.1453) (20.0505, -5.9559) (20.1469, -5.7776) knots 0 0 0 0 1 1 1 1
  spline S112 degree 3 poles (20.1469, -5.7776) (21.0651, -4.845) (22.1745, -4.3174) (23.4749, -4.1948) knots 0 0 0 0 1 1 1 1
  spline S113 degree 3 poles (23.4749, -4.1948) (23.8673, -3.5725) (24.2596, -2.9501) (24.6519, -2.3278) knots 0 0 0 0 1 1 1 1
  spline S114 degree 3 poles (24.6519, -2.3278) (25.318, -1.1172) (25.9945, 0.0868) (26.6812, 1.2843) knots 0 0 0 0 1 1 1 1
  spline S115 degree 3 poles (26.6812, 1.2843) (26.996, 1.7575) (27.3545, 2.1972) (27.7567, 2.6033) knots 0 0 0 0 1 1 1 1
  spline S116 degree 3 poles (27.7567, 2.6033) (28.3894, 3.1795) (29.1335, 3.423) (29.9889, 3.3339) knots 0 0 0 0 1 1 1 1
  spline S117 degree 3 poles (29.9889, 3.3339) (30.5331, 3.1815) (30.9457, 2.8636) (31.2268, 2.3801) knots 0 0 0 0 1 1 1 1
  spline S118 degree 3 poles (31.2268, 2.3801) (31.3301, 2.1673) (31.3437, 1.9508) (31.2674, 1.7308) knots 0 0 0 0 1 1 1 1
  spline S119 degree 3 poles (31.2674, 1.7308) (31.061, 1.5028) (30.8243, 1.469) (30.5571, 1.6293) knots 0 0 0 0 1 1 1 1
  spline S120 degree 3 poles (30.5571, 1.6293) (30.4671, 1.791) (30.3927, 1.9601) (30.3339, 2.1366) knots 0 0 0 0 1 1 1 1
  spline S121 degree 3 poles (30.3339, 2.1366) (30.0544, 2.4455) (29.7094, 2.547) (29.299, 2.441) knots 0 0 0 0 1 1 1 1
  spline S122 degree 3 poles (29.299, 2.441) (28.8702, 2.3503) (28.5117, 2.1406) (28.2235, 1.8119) knots 0 0 0 0 1 1 1 1
  spline S123 degree 3 poles (28.2235, 1.8119) (27.8963, 1.4415) (27.5986, 1.0491) (27.3306, 0.6349) knots 0 0 0 0 1 1 1 1
  spline S124 degree 3 poles (27.3306, 0.6349) (26.7386, -0.4002) (26.1568, -1.4419) (25.5854, -2.4902) knots 0 0 0 0 1 1 1 1
  spline S125 degree 3 poles (25.5854, -2.4902) (25.1829, -3.1464) (24.7703, -3.7958) (24.3475, -4.4383) knots 0 0 0 0 1 1 1 1
  spline S126 degree 3 poles (24.3475, -4.4383) (25.5575, -4.8706) (26.0378, -5.7093) (25.7883, -6.9546) knots 0 0 0 0 1 1 1 1
  spline S127 degree 3 poles (25.7883, -6.9546) (25.3369, -7.9894) (24.5455, -8.5644) (23.414, -8.6795) knots 0 0 0 0 1 1 1 1
  spline S128 degree 3 poles (23.414, -8.6795) (22.5987, -8.7342) (21.8073, -8.6191) (21.0398, -8.3345) knots 0 0 0 0 1 1 1 1
  spline S129 degree 3 poles (-25.7355, -0.8262) (-26.3008, -1.3291) (-26.9502, -1.6876) (-27.6836, -1.9017) knots 0 0 0 0 1 1 1 1
  spline S130 degree 3 poles (-27.6836, -1.9017) (-28.2465, -2.043) (-28.7133, -1.9009) (-29.0838, -1.4755) knots 0 0 0 0 1 1 1 1
  spline S131 degree 3 poles (-29.0838, -1.4755) (-29.111, -1.4214) (-29.1378, -1.3673) (-29.165, -1.3132) knots 0 0 0 0 1 1 1 1
  spline S132 degree 3 poles (-29.165, -1.3132) (-29.2364, -0.8962) (-29.1686, -0.5039) (-28.9621, -0.1362) knots 0 0 0 0 1 1 1 1
  spline S133 degree 3 poles (-28.9621, -0.1362) (-28.6325, 0.4008) (-28.2538, 0.9013) (-27.8257, 1.3655) knots 0 0 0 0 1 1 1 1
  spline S134 degree 3 poles (-27.8257, 1.3655) (-27.6808, 1.5471) (-27.5793, 1.75) (-27.5213, 1.9743) knots 0 0 0 0 1 1 1 1
  spline S135 degree 3 poles (-27.5213, 1.9743) (-28.0615, 1.9769) (-28.5619, 1.8349) (-29.0229, 1.5481) knots 0 0 0 0 1 1 1 1
  spline S136 degree 3 poles (-29.0229, 1.5481) (-29.5855, 1.1889) (-30.1131, 0.783) (-30.6058, 0.3305) knots 0 0 0 0 1 1 1 1
  spline S137 degree 3 poles (-30.6058, 0.3305) (-31.0843, 0.3189) (-31.2397, 0.5421) (-31.0725, 1.0002) knots 0 0 0 0 1 1 1 1
  spline S138 degree 3 poles (-31.0725, 1.0002) (-30.2673, 1.8528) (-29.3001, 2.4412) (-28.1706, 2.7657) knots 0 0 0 0 1 1 1 1
  spline S139 degree 3 poles (-28.1706, 2.7657) (-27.8865, 2.7928) (-27.6024, 2.7928) (-27.3183, 2.7657) knots 0 0 0 0 1 1 1 1
  spline S140 degree 3 poles (-27.3183, 2.7657) (-26.7538, 2.5485) (-26.5712, 2.1494) (-26.7704, 1.5684) knots 0 0 0 0 1 1 1 1
  spline S141 degree 3 poles (-26.7704, 1.5684) (-26.8715, 1.3388) (-26.9932, 1.1224) (-27.1357, 0.919) knots 0 0 0 0 1 1 1 1
  spline S142 degree 3 poles (-27.1357, 0.919) (-27.4912, 0.5366) (-27.8159, 0.1307) (-28.1098, -0.2985) knots 0 0 0 0 1 1 1 1
  spline S143 degree 3 poles (-28.1098, -0.2985) (-28.2104, -0.4664) (-28.2916, -0.6422) (-28.3533, -0.8262) knots 0 0 0 0 1 1 1 1
  spline S144 degree 3 poles (-28.3533, -0.8262) (-28.3841, -0.9182) (-28.3772, -1.0062) (-28.333, -1.09) knots 0 0 0 0 1 1 1 1
  spline S145 degree 3 poles (-28.333, -1.09) (-28.1434, -1.117) (-27.9543, -1.117) (-27.7648, -1.09) knots 0 0 0 0 1 1 1 1
  spline S146 degree 3 poles (-27.7648, -1.09) (-27.0821, -0.8262) (-26.4733, -0.4474) (-25.9384, 0.0464) knots 0 0 0 0 1 1 1 1
  spline S147 degree 3 poles (-25.9384, 0.0464) (-24.9822, 0.9481) (-24.1165, 1.9222) (-23.3409, 2.9686) knots 0 0 0 0 1 1 1 1
  spline S148 degree 3 poles (-23.3409, 2.9686) (-23.2687, 2.9668) (-23.2009, 2.9398) (-23.138, 2.8874) knots 0 0 0 0 1 1 1 1
  line L56 (-23.138, 2.8874) -> (-22.7119, 2.5425)
  spline S149 degree 3 poles (-22.7119, 2.5425) (-22.6847, 2.5019) (-22.6847, 2.4613) (-22.7119, 2.4207) knots 0 0 0 0 1 1 1 1
  spline S150 degree 3 poles (-22.7119, 2.4207) (-23.1599, 1.9049) (-23.593, 1.3773) (-24.0106, 0.8379) knots 0 0 0 0 1 1 1 1
  spline S151 degree 3 poles (-24.0106, 0.8379) (-24.3779, 0.3606) (-24.6482, -0.167) (-24.8223, -0.745) knots 0 0 0 0 1 1 1 1
  spline S152 degree 3 poles (-24.8223, -0.745) (-24.8613, -0.9102) (-24.841, -1.0658) (-24.7614, -1.2117) knots 0 0 0 0 1 1 1 1
  spline S153 degree 3 poles (-24.7614, -1.2117) (-24.4481, -1.2484) (-24.1506, -1.1943) (-23.8685, -1.0494) knots 0 0 0 0 1 1 1 1
  spline S154 degree 3 poles (-23.8685, -1.0494) (-23.2687, -0.7596) (-22.7005, -0.4214) (-22.1639, -0.0347) knots 0 0 0 0 1 1 1 1
  spline S155 degree 3 poles (-22.1639, -0.0347) (-21.638, 0.3693) (-21.1241, 0.7887) (-20.6217, 1.2234) knots 0 0 0 0 1 1 1 1
  spline S156 degree 3 poles (-20.6217, 1.2234) (-20.0032, 1.8691) (-19.3607, 2.4846) (-18.6939, 3.0701) knots 0 0 0 0 1 1 1 1
  spline S157 degree 3 poles (-18.6939, 3.0701) (-18.5449, 2.9483) (-18.3964, 2.8266) (-18.2474, 2.7048) knots 0 0 0 0 1 1 1 1
  spline S158 degree 3 poles (-18.2474, 2.7048) (-17.7502, 2.8778) (-17.2429, 2.9116) (-16.7254, 2.8063) knots 0 0 0 0 1 1 1 1
  spline S159 degree 3 poles (-16.7254, 2.8063) (-16.4641, 2.6936) (-16.2676, 2.5109) (-16.137, 2.2584) knots 0 0 0 0 1 1 1 1
  spline S160 degree 3 poles (-16.137, 2.2584) (-15.5955, 2.6689) (-14.9868, 2.9124) (-14.3106, 2.9889) knots 0 0 0 0 1 1 1 1
  spline S161 degree 3 poles (-14.3106, 2.9889) (-13.3978, 2.9757) (-12.8227, 2.5292) (-12.5857, 1.6496) knots 0 0 0 0 1 1 1 1
  spline S162 degree 3 poles (-12.5857, 1.6496) (-11.7748, 2.1903) (-10.8953, 2.5758) (-9.9476, 2.8063) knots 0 0 0 0 1 1 1 1
  spline S163 degree 3 poles (-9.9476, 2.8063) (-9.2974, 2.9375) (-8.6477, 2.9375) (-7.9995, 2.8063) knots 0 0 0 0 1 1 1 1
  spline S164 degree 3 poles (-7.9995, 2.8063) (-7.648, 2.6849) (-7.3842, 2.4617) (-7.2081, 2.1366) knots 0 0 0 0 1 1 1 1
  spline S165 degree 3 poles (-7.2081, 2.1366) (-6.454, 2.5847) (-5.6489, 2.9027) (-4.7931, 3.0904) knots 0 0 0 0 1 1 1 1
  spline S166 degree 3 poles (-4.7931, 3.0904) (-4.0331, 3.1844) (-3.6137, 2.8529) (-3.5349, 2.096) knots 0 0 0 0 1 1 1 1
  spline S167 degree 3 poles (-3.5349, 2.096) (-3.5916, 1.662) (-3.7337, 1.2562) (-3.9611, 0.8785) knots 0 0 0 0 1 1 1 1
  spline S168 degree 3 poles (-3.9611, 0.8785) (-4.3387, 0.2651) (-4.7513, -0.3234) (-5.1989, -0.887) knots 0 0 0 0 1 1 1 1
  spline S169 degree 3 poles (-5.1989, -0.887) (-4.9418, -0.9344) (-4.6848, -0.9818) (-4.4278, -1.0291) knots 0 0 0 0 1 1 1 1
  spline S170 degree 3 poles (-4.4278, -1.0291) (-4.2269, -0.8067) (-4.0443, -0.5632) (-3.8799, -0.2985) knots 0 0 0 0 1 1 1 1
  line L57 (-3.8799, -0.2985) -> (-3.1493, 0.5943)
  spline S171 degree 3 poles (-3.1493, 0.5943) (-2.557, 1.2244) (-1.9008, 1.7723) (-1.1809, 2.2381) knots 0 0 0 0 1 1 1 1
  spline S172 degree 3 poles (-1.1809, 2.2381) (-0.8389, 2.4226) (-0.4872, 2.585) (-0.1257, 2.7251) knots 0 0 0 0 1 1 1 1
  spline S173 degree 3 poles (-0.1257, 2.7251) (0.2786, 2.8306) (0.6845, 2.8441) (1.0919, 2.7657) knots 0 0 0 0 1 1 1 1
  spline S174 degree 3 poles (1.0919, 2.7657) (1.3711, 2.5944) (1.5132, 2.3441) (1.518, 2.0149) knots 0 0 0 0 1 1 1 1
  spline S175 degree 3 poles (1.518, 2.0149) (2.282, 2.716) (3.1816, 3.0204) (4.217, 2.928) knots 0 0 0 0 1 1 1 1
  spline S176 degree 3 poles (4.217, 2.928) (4.858, 2.7604) (5.2707, 2.3613) (5.4548, 1.7308) knots 0 0 0 0 1 1 1 1
  spline S177 degree 3 poles (5.4548, 1.7308) (6.3534, 2.3301) (7.2936, 2.8645) (8.2756, 3.3339) knots 0 0 0 0 1 1 1 1
  spline S178 degree 3 poles (8.2756, 3.3339) (9.013, 4.613) (9.9058, 5.7764) (10.9542, 6.8243) knots 0 0 0 0 1 1 1 1
  spline S179 degree 3 poles (10.9542, 6.8243) (11.3533, 7.1958) (11.8133, 7.4664) (12.3341, 7.636) knots 0 0 0 0 1 1 1 1
  spline S180 degree 3 poles (12.3341, 7.636) (13.1638, 7.7801) (13.5629, 7.4351) (13.5314, 6.601) knots 0 0 0 0 1 1 1 1
  spline S181 degree 3 poles (13.5314, 6.601) (13.4524, 6.3349) (13.3307, 6.0914) (13.1661, 5.8705) knots 0 0 0 0 1 1 1 1
  spline S182 degree 3 poles (13.1661, 5.8705) (12.8347, 5.4849) (12.4762, 5.1264) (12.0906, 4.795) knots 0 0 0 0 1 1 1 1
  spline S183 degree 3 poles (12.0906, 4.795) (11.1036, 4.0387) (10.0619, 3.3622) (8.9655, 2.7657) knots 0 0 0 0 1 1 1 1
  spline S184 degree 3 poles (8.9655, 2.7657) (8.8753, 2.6594) (8.8145, 2.5445) (8.7829, 2.4207) knots 0 0 0 0 1 1 1 1
  spline S185 degree 3 poles (8.7829, 2.4207) (9.4149, 2.8072) (10.0981, 2.9493) (10.8325, 2.8469) knots 0 0 0 0 1 1 1 1
  spline S186 degree 3 poles (10.8325, 2.8469) (11.3953, 2.7169) (11.7403, 2.3719) (11.8674, 1.8119) knots 0 0 0 0 1 1 1 1
  spline S187 degree 3 poles (11.8674, 1.8119) (12.4436, 2.2658) (13.0862, 2.5972) (13.7952, 2.8063) knots 0 0 0 0 1 1 1 1
  spline S188 degree 3 poles (13.7952, 2.8063) (14.1315, 2.8653) (14.4697, 2.8788) (14.8099, 2.8469) knots 0 0 0 0 1 1 1 1
  spline S189 degree 3 poles (14.8099, 2.8469) (15.1554, 2.7719) (15.4057, 2.5757) (15.5607, 2.2584) knots 0 0 0 0 1 1 1 1
  spline S190 degree 3 poles (15.5607, 2.2584) (16.0968, 2.682) (16.7056, 2.9255) (17.3871, 2.9889) knots 0 0 0 0 1 1 1 1
  spline S191 degree 3 poles (17.3871, 2.9889) (18.5386, 2.9198) (19.0932, 2.311) (19.0511, 1.1626) knots 0 0 0 0 1 1 1 1
  spline S192 degree 3 poles (19.0511, 1.1626) (18.9093, 0.6489) (18.6522, 0.2024) (18.2799, -0.1768) knots 0 0 0 0 1 1 1 1
  spline S193 degree 3 poles (18.2799, -0.1768) (17.4808, -0.9859) (16.5406, -1.5744) (15.4592, -1.9423) knots 0 0 0 0 1 1 1 1
  spline S194 degree 3 poles (15.4592, -1.9423) (14.7726, -2.1501) (14.0962, -2.1231) (13.4299, -1.8611) knots 0 0 0 0 1 1 1 1
  spline S195 degree 3 poles (13.4299, -1.8611) (12.9721, -1.5926) (12.7624, -1.1935) (12.8009, -0.6638) knots 0 0 0 0 1 1 1 1
  spline S196 degree 3 poles (12.8009, -0.6638) (12.6002, -0.8751) (12.3635, -0.936) (12.0906, -0.8464) knots 0 0 0 0 1 1 1 1
  spline S197 degree 3 poles (12.0906, -0.8464) (11.82, -0.6164) (11.82, -0.3865) (12.0906, -0.1565) knots 0 0 0 0 1 1 1 1
  spline S198 degree 3 poles (12.0906, -0.1565) (12.9639, 0.3379) (13.7688, 0.9264) (14.5055, 1.609) knots 0 0 0 0 1 1 1 1
  spline S199 degree 3 poles (14.5055, 1.609) (14.5965, 1.7135) (14.6709, 1.8285) (14.7287, 1.954) knots 0 0 0 0 1 1 1 1
  spline S200 degree 3 poles (14.7287, 1.954) (14.7123, 1.9923) (14.6852, 2.0194) (14.6475, 2.0351) knots 0 0 0 0 1 1 1 1
  spline S201 degree 3 poles (14.6475, 2.0351) (14.2054, 2.0739) (13.786, 1.9927) (13.3894, 1.7916) knots 0 0 0 0 1 1 1 1
  spline S202 degree 3 poles (13.3894, 1.7916) (12.685, 1.4428) (12.056, 0.9897) (11.5021, 0.432) knots 0 0 0 0 1 1 1 1
  spline S203 degree 3 poles (11.5021, 0.432) (10.8474, -0.7367) (9.9071, -1.5958) (8.6814, -2.1452) knots 0 0 0 0 1 1 1 1
  spline S204 degree 3 poles (8.6814, -2.1452) (8.1756, -2.2085) (7.9998, -1.9988) (8.1538, -1.5161) knots 0 0 0 0 1 1 1 1
  spline S205 degree 3 poles (8.1538, -1.5161) (8.8418, -1.2026) (9.4574, -0.7832) (10.0004, -0.258) knots 0 0 0 0 1 1 1 1
  line L58 (10.0004, -0.258) -> (10.6092, 0.5132)
  spline S206 degree 3 poles (10.6092, 0.5132) (10.7757, 0.7957) (10.911, 1.0934) (11.0151, 1.4061) knots 0 0 0 0 1 1 1 1
  spline S207 degree 3 poles (11.0151, 1.4061) (11.1056, 1.7325) (10.9907, 1.9422) (10.6701, 2.0351) knots 0 0 0 0 1 1 1 1
  spline S208 degree 3 poles (10.6701, 2.0351) (10.3976, 2.064) (10.127, 2.0505) (9.8584, 1.9946) knots 0 0 0 0 1 1 1 1
  spline S209 degree 3 poles (9.8584, 1.9946) (9.1369, 1.7321) (8.4808, 1.36) (7.89, 0.8785) knots 0 0 0 0 1 1 1 1
  spline S210 degree 3 poles (7.89, 0.8785) (7.4165, 0.0126) (6.943, -0.8532) (6.4695, -1.719) knots 0 0 0 0 1 1 1 1
  spline S211 degree 3 poles (6.4695, -1.719) (6.199, -2.0742) (5.854, -2.1756) (5.4345, -2.0234) knots 0 0 0 0 1 1 1 1
  spline S212 degree 3 poles (5.4345, -2.0234) (5.1615, -1.795) (5.0735, -1.5041) (5.1707, -1.1508) knots 0 0 0 0 1 1 1 1
  spline S213 degree 3 poles (5.1707, -1.1508) (5.3537, -0.6163) (5.6378, -0.1428) (6.023, 0.2697) knots 0 0 0 0 1 1 1 1
  spline S214 degree 3 poles (6.023, 0.2697) (6.4045, 0.6782) (6.8103, 1.057) (7.2406, 1.4061) knots 0 0 0 0 1 1 1 1
  spline S215 degree 3 poles (7.2406, 1.4061) (7.3732, 1.6171) (7.4815, 1.8336) (7.5653, 2.0554) knots 0 0 0 0 1 1 1 1
  spline S216 degree 3 poles (7.5653, 2.0554) (6.7903, 1.6445) (6.053, 1.1777) (5.3534, 0.6552) knots 0 0 0 0 1 1 1 1
  spline S217 degree 3 poles (5.3534, 0.6552) (4.5999, -0.3711) (3.6529, -1.1693) (2.5124, -1.7393) knots 0 0 0 0 1 1 1 1